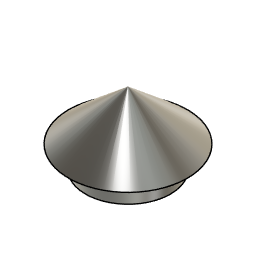
wind_top_cover (Autodesk Fusion 360 design; units mm, degrees)
Autodesk Fusion 360 part; units mm, degrees
note: some values were not read from the file. Set by a fixed rule: which sketch regions a step uses.
sketch "Szkic1" plane through (0, 0, 0) normal (0, 1, 0) x (1, 0, 0)
  line L0 (-6, 0) -> (0, -5.0346)
  line L1 (0, -3.3564) -> (0, -5.0346)
  line L2 (-2.5, 0) -> (1.3455, 0) construction
  line L3 (-2.5, 0) -> (0, -2.0977)
  line L4 (-2.5, 0) -> (1.1341, 0) construction
  line L5 (0, -2.0977) -> (0, -5.0346)
  line L6 (-2.5, 0) -> (-4, 1.2586)
  line L7 (-6, 0) -> (-4, 0) construction
  line L8 (-2.5, 0) -> (3.6054, 0) construction
  line L9 (-6, 0) -> (-8.0308, 1.704)
  line L10 (-8.0308, 1.704) -> (-6, 1.704)
  line L11 (-6, 1.704) -> (-5.75, 4.704)
  line L12 (-5.75, 4.704) -> (-4, 4.704)
  line L13 (-4, 4.704) -> (-4, 1.2586)
  dimension "d4" = 6
  dimension "d5" = 40
  dimension "d7" = 40
  dimension "d11" = 2
  dimension "d13" = 4
  dimension "d14" = 1.75
  dimension "d15" = 3
  constraint horizontal L7
  constraint perpendicular L1 L7
  constraint horizontal L2
  constraint coincident L2.start L7
  constraint horizontal L4
  constraint parallel L1 L5
  constraint parallel L3 L6
  constraint collinear L7 L8
  constraint parallel L0 L9
  constraint perpendicular L12 L13
  constraint vertical L13
  measures "d4" distance of origin L0.start
  measures "d5" angle of L0 L7
  measures "d7" angle of L3 L4
  measures "d11" horizontal distance of L6.end L10.end
  measures "d13" distance of origin L13
  measures "d14" distance of L11.end L12.end
  measures "d15" vertical distance of L10.end L11.end
revolve "Obrót1" add sketch "Szkic1" angle 360 about axis through (0, 0, 1.75) along (0, 0, 1)
